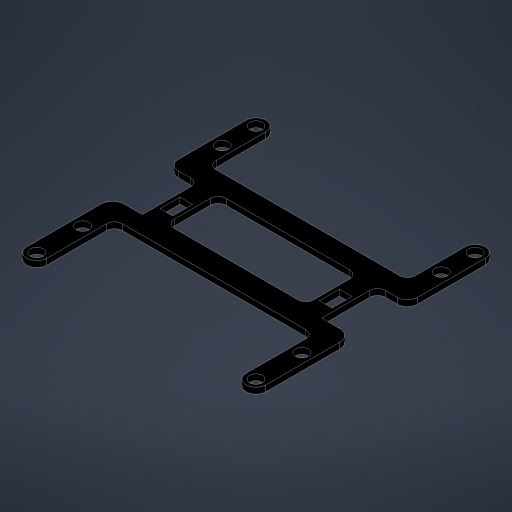
# Autodesk Inventor part: HandleHolder_V2-Carbon
Saved by Autodesk Inventor 2023 (Build 270158000, 158)
## iProperties
Created: 2023-04-10
Part Number: HandleHolder_V2-Carbon
Material: Generic
Document SubType Name: Modeling
Designer: Elias Braun
Density: 1 g/cm^3
Appearance: Default
Author: Elias Braun
Autodesk Inventor part; units mm, degrees
ref_plane "YZ Plane" through (0, 0, 0) normal (1, 0, 0) x (0, 1, 0)
ref_plane "XZ Plane" through (0, 0, 0) normal (0, 1, 0) x (-1, 0, 0)
ref_plane "XY Plane" through (0, 0, 0) normal (0, 0, 1) x (1, 0, 0)
sketch "Sketch1" plane through (0, 0, 0) normal (0, 1, 0) x (-1, 0, 0)
  line L0 (0, 0) -> (0, -5.5344) construction
  line L1 (0, 0) -> (-3.3399, 0) construction
  arc A0 (27.5, 8) -> (30, 10.5) centre (27.5, 10.5) ccw
  arc A1 (-30, 10.5) -> (-27.5, 8) centre (-27.5, 10.5) ccw
  line L2 (25, 13) -> (-25, 13)
  line L3 (22.5, 8) -> (27.5, 8)
  line L4 (-27.5, 8) -> (-22.5, 8)
  line L5 (-17.5, 0) -> (-20, 0) construction
  line L6 (17.5, 8) -> (-17.5, 8)
  line L7 (17.5, 8) -> (-17.5, 8)
  circle A2 centre (27.5, 27.5) radius 1.6
  circle A3 centre (-27.5, 27.5) radius 1.6
  line L8 (0, 0) -> (0, 8) construction
  arc A4 (30, 27.5) -> (25, 27.5) centre (27.5, 27.5) ccw
  line L9 (30, 27.5) -> (30, 10.5)
  line L10 (25, 13) -> (25, 27.5)
  arc A5 (-25, 27.5) -> (-30, 27.5) centre (-27.5, 27.5) ccw
  line L11 (-30, 27.5) -> (-30, 10.5)
  line L12 (-25, 13) -> (-25, 27.5)
  line L13 (27.5, 27.5) -> (27.5, 16) construction
  circle A6 centre (27.5, 16) radius 1.6
  circle A7 centre (-27.5, 16) radius 1.6
  arc A8 (30, -10.5) -> (27.5, -8) centre (27.5, -10.5) ccw
  arc A9 (-27.5, -8) -> (-30, -10.5) centre (-27.5, -10.5) ccw
  line L14 (25, -13) -> (-25, -13)
  line L15 (22.5, -8) -> (27.5, -8)
  line L16 (-27.5, -8) -> (-22.5, -8)
  line L17 (17.5, -8) -> (-17.5, -8)
  line L18 (17.5, -8) -> (-17.5, -8)
  circle A10 centre (27.5, -27.5) radius 1.6
  circle A11 centre (-27.5, -27.5) radius 1.6
  arc A12 (25, -27.5) -> (30, -27.5) centre (27.5, -27.5) ccw
  line L19 (30, -27.5) -> (30, -10.5)
  line L20 (25, -13) -> (25, -27.5)
  line L21 (-25, -13) -> (-25, -27.5)
  line L22 (-30, -27.5) -> (-30, -10.5)
  arc A13 (-30, -27.5) -> (-25, -27.5) centre (-27.5, -27.5) ccw
  circle A14 centre (27.5, -16) radius 1.6
  circle A15 centre (-27.5, -16) radius 1.6
  line L23 (22.5, -8) -> (22.5, 8)
  line L24 (17.5, 8) -> (17.5, -8)
  line L25 (-17.5, -8) -> (-17.5, 8)
  line L26 (-22.5, 8) -> (-22.5, -8)
  line L27 (27.5, -16) -> (27.5, -19)
  circle A16 centre (27.5, -19) radius 1.6
  circle A17 centre (-27.5, -19) radius 1.6
  line L28 (18.4125, 2.5) -> (18.4125, -2.5)
  line L29 (18.4125, -2.5) -> (21.5875, -2.5)
  line L30 (21.5875, -2.5) -> (21.5875, 2.5)
  line L31 (21.5875, 2.5) -> (18.4125, 2.5)
  line L32 (18.4125, 2.5) -> (21.5875, -2.5) construction
  line L33 (18.4125, -2.5) -> (21.5875, 2.5) construction
  line L34 (-18.4125, 2.5) -> (-18.4125, -2.5)
  line L35 (-18.4125, -2.5) -> (-21.5875, -2.5)
  line L36 (-21.5875, -2.5) -> (-21.5875, 2.5)
  line L37 (-21.5875, 2.5) -> (-18.4125, 2.5)
  line L38 (-18.4125, 2.5) -> (-21.5875, -2.5) construction
  line L39 (-18.4125, -2.5) -> (-21.5875, 2.5) construction
  point P0 (20, 0)
  point P1 (0, -8)
  dimension "d41" = 8
  dimension "d44" = 11.5
  dimension "d45" = 3.2
  dimension "d66" = 3
  dimension "d67" = 3.2
  dimension "d68" = 5
  dimension "d69" = 3.175
  dimension "d70" = 5
  dimension "d71" = 3.175
  constraints: 80 end point, 29 symmetric about line, 18 centre point, 16 point on circle, 9 vertical, 7 parallel, 4 midpoint, 3 coincident, 2 horizontal, 2 perpendicular, 11 other
  measures "d41" distance of L0.start L8.end
  measures "d44" distance of L13.start L13.end
  measures "d45" diameter of A6
  measures "d66" distance of L27.start L27.end
  measures "d67" diameter of A16
  measures "d68" distance of L28.start L28.end
  measures "d69" distance of L29.end L28.end
  measures "d70" distance of L34.start L34.end
  measures "d71" distance of L34.end L35.end
extrude "Extrusion1" add sketch "Sketch1" along normal blind 1.5 contours L3 L23 L15 A8 L19 A12 L20 L14 L21 A13 L22 A9 L16 L26 L4 A1 L11 A5 L12 L2 L10 A4 L9 A0 | A14 A16 | A15 A17 picked at (27.4973, -15.4078) picked at (-27.5657, -15.4115)
fillet "Fillet1" radius 2 6 edges at (22.5, 0.75, 8) (-22.5, 0.75, 8) (-17.5, 0.75, 8) (17.5, 0.75, 8) (-25, 0.75, 13) (25, 0.75, 13)
sketch "Sketch5" plane through (0, 1.5, 0) normal (0, 1, 0) x (1, 0, 0)
  arc A0 (-23, -13) -> (-25, -15) centre (-23, -15) ccw projected
  line L0 (-25, -15) -> (25, -15)
  line L1 (25, -15) -> (25, -10.5)
  line L2 (25, -10.5) -> (-25, -10.5)
  line L3 (-25, -10.5) -> (-25, -15)
  arc A1 (-17.5, -6) -> (-15.5, -8) centre (-15.5, -6) ccw projected
  line L4 (-17.5, -6) -> (17.5, -6)
  line L5 (17.5, -6) -> (17.5, -8)
  line L6 (17.5, -8) -> (-17.5, -8)
  line L7 (-17.5, -8) -> (-17.5, -6)
  line L8 (-17.5, -6) -> (17.5, -6)
  line L9 (17.5, -6) -> (17.5, -5)
  line L10 (17.5, -5) -> (-17.5, -5)
  line L11 (-17.5, -5) -> (-17.5, -6)
  line L12 (-17.5, 16.5) -> (17.5, 16.5)
  line L13 (17.5, 16.5) -> (17.5, 18.5)
  line L14 (17.5, 18.5) -> (-17.5, 18.5)
  line L15 (-17.5, 18.5) -> (-17.5, 16.5)
  point P0 (0, 0)
  point P1 (17.5, -6)
  dimension "d49" = 50
  dimension "d50" = 4.5
  dimension "d56" = 2
  dimension "d57" = 35
  dimension "d58" = 1
  dimension "d59" = 35
  dimension "d60" = 2
  constraints: 32 end point, 8 parallel, 4 horizontal, 4 perpendicular
  measures "d49" distance of L2.end L1.end
  measures "d50" distance of L1.end L0.end
  measures "d56" distance of L4.end L5.end
  measures "d57" distance of L10.end L9.end
  measures "d58" distance of L9.end L8.end
  measures "d59" distance of L14.end L13.end
  measures "d60" distance of L13.end L12.end
extrude "Extrusion6" cut sketch "Sketch5" against normal blind 1.5 contours L3 L2 L1 L0
extrude "Extrusion7" add sketch "Sketch5" against normal blind 1.5 contours L4 L5 L6 A1 | L11 L10 L9 L4 | A1 L6 L7
fillet "Fillet5" radius 2 10 edges at (-25, 0.75, 10.5) (25, 0.75, 10.5) (22.5, 0.75, -8) (17.5, 0.75, -8) (17.5, 0.75, 5) (-17.5, 0.75, 5) (-17.5, 0.75, -8) (-22.5, 0.75, -8) (25, 0.75, -13) (-25, 0.75, -13)
sketch "Sketch6" plane through (0, 1.5, 0) normal (0, 1, 0) x (1, 0, 0)
  line L0 (-30, -10.5) -> (-30, -27.5) projected
  arc A0 (-24.5, -8) -> (-22.5, -6) centre (-24.5, -6) ccw projected
  line L1 (-30, -10.5) -> (-22.5, -10.5)
  line L2 (-22.5, -10.5) -> (-22.5, -6)
  line L3 (-22.5, -6) -> (-30, -6)
  line L4 (-30, -6) -> (-30, -10.5)
  line L5 (30, -27.5) -> (30, -10.5) projected
  line L6 (22.4338, -6) -> (30, -6)
  line L7 (30, -6) -> (30, -10.5)
  line L8 (30, -10.5) -> (22.4338, -10.5)
  line L9 (22.4338, -10.5) -> (22.4338, -6)
  arc A1 (27.5, 18.5) -> (30, 21) centre (27.5, 21) ccw projected
  arc A2 (24.5, 18.5) -> (22.5, 16.5) centre (24.5, 16.5) ccw projected
  line L10 (30, 21) -> (22.5, 21)
  line L11 (22.5, 21) -> (22.5, 16.5)
  line L12 (22.5, 16.5) -> (30, 16.5)
  line L13 (30, 16.5) -> (30, 21)
  arc A3 (-30, 21) -> (-27.5, 18.5) centre (-27.5, 21) ccw projected
  line L14 (-30, 21) -> (-22.5, 21)
  line L15 (-22.5, 21) -> (-22.5, 16.5)
  line L16 (-22.5, 16.5) -> (-30, 16.5)
  line L17 (-30, 16.5) -> (-30, 21)
  point P0 (0, 0)
  constraints: 32 end point, 8 parallel, 4 horizontal, 4 perpendicular, 3 point on line
extrude "Extrusion8" add sketch "Sketch6" against normal blind 1.5 contours L4 L3 L2 L1 | L6 L7 L8 L9
fillet "Fillet6" radius 3 2 edges at (30, 0.75, 6) (-30, 0.75, 6)
body "Solid1"
